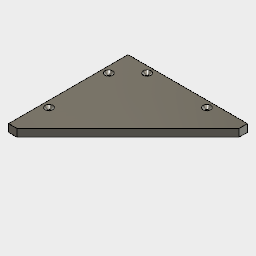
Full Assembly (Autodesk Fusion 360 archive; units mm, degrees)
design "Joining Plate (90 Degree)"
Autodesk Fusion 360 part; units mm, degrees
sketch "Sketch1" plane through (0, 0, 0) normal (0, 1, 0) x (1, 0, 0)
  line L0 (0, 0) -> (140, 0)
  line L1 (140, -10) -> (10, -140)
  line L2 (0, -140) -> (0, 0)
  line L3 (140, 0) -> (140, -10)
  line L4 (0, -140) -> (10, -140)
  circle A0 centre (30, -7.5) radius 1.5
  circle A1 centre (100, -7.5) radius 1.5
  circle A2 centre (7.5, -30) radius 1.5
  circle A3 centre (7.5, -100) radius 1.5
  dimension "d5" = 10
  dimension "d6" = 10
  dimension "d7" = 140
  dimension "d8" = 140
  dimension "d9" = 3
  dimension "d10" = 3
  dimension "d11" = 3
  dimension "d12" = 3
  dimension "d13" = 7.5
  dimension "d14" = 7.5
  dimension "d15" = 7.5
  dimension "d16" = 7.5
  dimension "d17" = 30
  dimension "d18" = 100
  dimension "d19" = 30
  dimension "d20" = 100
  measures "d5" distance of L0.end L1.start
  measures "d6" distance of L2.start L1.end
  measures "d7" distance of L0.start L2.start
  measures "d8" distance of L0.start L0.end
  measures "d9" diameter of A0
  measures "d10" diameter of A1
  measures "d11" diameter of A2
  measures "d12" diameter of A3
  measures "d13" distance of L0 A0.centre
  measures "d14" distance of L0 A1.centre
  measures "d15" distance of L2 A2.centre
  measures "d16" distance of L2 A3.centre
  measures "d17" distance of L0 A2.centre
  measures "d18" distance of L0 A3.centre
  measures "d19" distance of L2 A0.centre
  measures "d20" distance of L2 A1.centre
extrude "Extrude1" add sketch "Sketch1" along normal blind 9
chamfer "Chamfer1" distance 3 angle 45 4 edges at (28.6015, 9, 6.9576) (6.1015, 9, 29.4576) (98.6015, 9, 6.9576) (6.1015, 9, 99.4576)

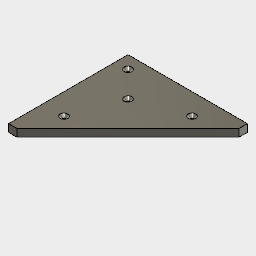
design "Joining Plate (180 Degree)"
Autodesk Fusion 360 part; units mm, degrees
sketch "Sketch1" plane through (0, 0, 0) normal (0, 1, 0) x (1, 0, 0)
  line L0 (0, 0) -> (140, 0)
  line L1 (140, -10) -> (10, -140)
  line L2 (0, -140) -> (0, 0)
  line L3 (140, 0) -> (140, -10)
  line L4 (0, -140) -> (10, -140)
  circle A0 centre (15, -15) radius 1.5
  circle A1 centre (100, -25) radius 1.5
  circle A2 centre (45, -45) radius 1.5
  circle A3 centre (25, -100) radius 1.5
  dimension "d5" = 10
  dimension "d6" = 10
  dimension "d7" = 140
  dimension "d8" = 140
  dimension "d9" = 3
  dimension "d10" = 3
  dimension "d11" = 3
  dimension "d12" = 3
  dimension "d26" = 45
  dimension "d27" = 45
  dimension "d28" = 15
  dimension "d29" = 15
  dimension "d30" = 25
  dimension "d31" = 25
  dimension "d32" = 100
  dimension "d33" = 100
  measures "d5" distance of L0.end L1.start
  measures "d6" distance of L2.start L1.end
  measures "d7" distance of L0.start L2.start
  measures "d8" distance of L0.start L0.end
  measures "d9" diameter of A0
  measures "d10" diameter of A1
  measures "d11" diameter of A2
  measures "d12" diameter of A3
  measures "d26" distance of L2 A2.centre
  measures "d27" distance of L0 A2.centre
  measures "d28" distance of L0 A0.centre
  measures "d29" distance of L2 A0.centre
  measures "d30" distance of L2 A3.centre
  measures "d31" distance of L0 A1.centre
  measures "d32" distance of L2 A1.centre
  measures "d33" distance of L0 A3.centre
extrude "Extrude1" add sketch "Sketch1" along normal blind 9
chamfer "Chamfer1" distance 3 angle 45 4 edges at (13.6015, 9, 14.4576) (43.6015, 9, 44.4576) (98.6015, 9, 24.4576) (23.6015, 9, 99.4576)

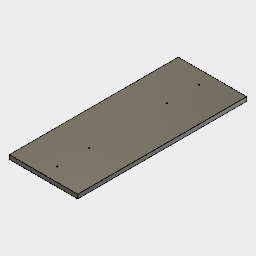
design "Gantry Foot Plate"
Autodesk Fusion 360 part; units mm, degrees
sketch "Sketch1" plane through (0, 0, 0) normal (0, 1, 0) x (1, 0, 0)
  line L0 (0, 0) -> (150, 0)
  line L1 (150, 0) -> (150, -370)
  line L2 (150, -370) -> (0, -370)
  line L3 (0, -370) -> (0, 0)
  line L4 (75, 0) -> (75, -370) construction
  circle A0 centre (75, -30) radius 1.5
  circle A1 centre (75, -100) radius 1.5
  circle A2 centre (75, -270) radius 1.5
  circle A3 centre (75, -340) radius 1.5
  dimension "d1" = 150
  dimension "d2" = 370
  dimension "d3" = 3
  dimension "d4" = 3
  dimension "d5" = 3
  dimension "d6" = 3
  dimension "d7" = 30
  dimension "d8" = 100
  dimension "d9" = 30
  dimension "d10" = 100
  measures "d1" distance of L0.start L0.end
  measures "d2" distance of L0.start L2.end
  measures "d3" diameter of A2
  measures "d4" diameter of A3
  measures "d5" diameter of A1
  measures "d6" diameter of A0
  measures "d7" distance of L0 A0.centre
  measures "d8" distance of L0 A1.centre
  measures "d9" distance of L2 A3.centre
  measures "d10" distance of L2 A2.centre
extrude "Extrude1" add sketch "Sketch1" along normal blind 9
chamfer "Chamfer1" distance 3 angle 45 4 edges at (73.6015, 0, 339.4576) (73.6015, 0, 269.4576) (73.6015, 0, 99.4576) (73.6015, 0, 29.4576)

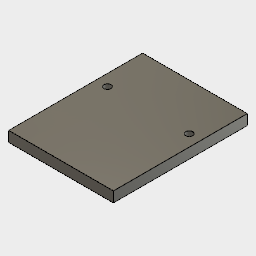
design "Gantry Mount Plate"
Autodesk Fusion 360 part; units mm, degrees
sketch "Sketch1" plane through (0, 0, 0) normal (0, 1, 0) x (1, 0, 0)
  line L0 (0, 0) -> (90, 0)
  line L1 (90, 0) -> (90, -115)
  line L2 (90, -115) -> (0, -115)
  line L3 (0, -115) -> (0, 0)
  dimension "d1" = 90
  dimension "d2" = 115
  measures "d1" distance of L0.start L0.end
  measures "d2" distance of L0.start L2.end
sketch "Sketch2" plane through (0, 0, 0) normal (0, 1, 0) x (1, 0, 0)
  circle A0 centre (10, -40) radius 3
  circle A1 centre (80, -40) radius 3
  line L0 (0, 0) -> (90, 0)
  line L1 (0, -115) -> (0, 0)
  line L2 (90, 0) -> (90, -115)
  dimension "d3" = 6
  dimension "d4" = 6
  dimension "d5" = 40
  dimension "d6" = 40
  dimension "d7" = 10
  dimension "d8" = 10
  measures "d3" diameter of A0
  measures "d4" diameter of A1
  measures "d5" distance of A0.centre L0
  measures "d6" distance of A1.centre L0
  measures "d7" distance of A0.centre L1
  measures "d8" distance of A1.centre L2
extrude "Extrude1" add sketch "Sketch1" along normal blind 9
extrude "Extrude2" cut sketch "Sketch2" along normal blind 9

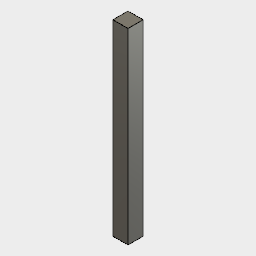
design "Gantry Base Beam"
Autodesk Fusion 360 part; units mm, degrees
sketch "Sketch1" plane through (0, 0, 0) normal (0, 1, 0) x (1, 0, 0)
  line L0 (0, 0) -> (30, 0)
  line L1 (30, 0) -> (30, -30)
  line L2 (30, -30) -> (0, -30)
  line L3 (0, -30) -> (0, 0)
  dimension "d1" = 30
  dimension "d2" = 30
  measures "d1" distance of L0.start L0.end
  measures "d2" distance of L0.start L2.end
extrude "Extrude1" add sketch "Sketch1" along normal blind 370

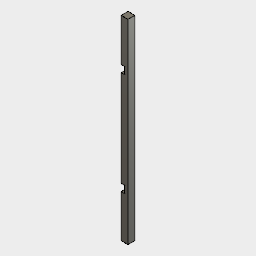
design "Frame Horizontal Beam"
Autodesk Fusion 360 part; units mm, degrees
sketch "Sketch1" plane through (0, 0, 0) normal (0, 1, 0) x (1, 0, 0)
  line L0 (0, 0) -> (30, 0)
  line L1 (30, 0) -> (30, -30)
  line L2 (30, -30) -> (0, -30)
  line L3 (0, -30) -> (0, 0)
  dimension "d1" = 30
  dimension "d2" = 30
  measures "d1" distance of L0.start L0.end
  measures "d2" distance of L0.start L2.end
extrude "Extrude1" add sketch "Sketch1" along normal blind 846
sketch "Sketch2" plane through (0, 0, 0) normal (-1, 0, 0) x (0, 0, 1)
  line L0 (0, 0) -> (30, 0)
  line L1 (30, 0) -> (30, 846)
  line L2 (30, 846) -> (0, 846)
  line L3 (0, 846) -> (0, 0)
  line L4 (0, 215) -> (30, 215)
  line L5 (30, 215) -> (30, 185)
  line L6 (30, 185) -> (0, 185)
  line L7 (0, 185) -> (0, 215)
  line L8 (0, 631) -> (30, 631)
  line L9 (30, 631) -> (30, 661)
  line L10 (30, 661) -> (0, 661)
  line L11 (0, 661) -> (0, 631)
  dimension "d5" = 30
  dimension "d6" = 30
  dimension "d7" = 185
  dimension "d8" = 185
  dimension "d9" = 380
  measures "d5" distance of L8.start L10.end
  measures "d6" distance of L4.end L5.end
  measures "d7" distance of L0 L6
  measures "d8" distance of L2 L10
extrude "Extrude2" cut sketch "Sketch2" against normal blind 15 contours L1 L3 L4 L5 L6 L7 | L1 L3 L8 L9 L10 L11

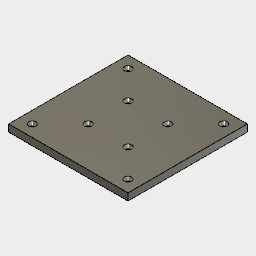
design "Joining Plate (360 Degrees)"
Autodesk Fusion 360 part; units mm, degrees
sketch "Sketch1" plane through (0, 0, 0) normal (0, 1, 0) x (1, 0, 0)
  line L0 (0, 0) -> (150, 0)
  line L1 (150, 0) -> (150, -150)
  line L2 (150, -150) -> (0, -150)
  line L3 (0, -150) -> (0, 0)
  circle A0 centre (15, -15) radius 1.5
  circle A1 centre (135, -15) radius 1.5
  circle A2 centre (135, -135) radius 1.5
  circle A3 centre (15, -135) radius 1.5
  circle A4 centre (50, -100) radius 1.5
  circle A5 centre (50, -50) radius 1.5
  circle A6 centre (100, -50) radius 1.5
  circle A7 centre (100, -100) radius 1.5
  dimension "d1" = 150
  dimension "d2" = 150
  dimension "d3" = 3
  dimension "d4" = 3
  dimension "d5" = 3
  dimension "d6" = 3
  dimension "d7" = 3
  dimension "d8" = 3
  dimension "d9" = 3
  dimension "d10" = 3
  dimension "d12" = 15
  dimension "d14" = 15
  dimension "d15" = 15
  dimension "d16" = 15
  dimension "d17" = 15
  dimension "d18" = 15
  dimension "d19" = 15
  dimension "d20" = 15
  dimension "d21" = 50
  dimension "d22" = 50
  dimension "d23" = 50
  dimension "d24" = 50
  dimension "d25" = 50
  dimension "d26" = 50
  dimension "d27" = 50
  dimension "d28" = 50
  measures "d1" distance of L0.start L0.end
  measures "d2" distance of L0.start L2.end
  measures "d3" diameter of A0
  measures "d4" diameter of A1
  measures "d5" diameter of A2
  measures "d6" diameter of A3
  measures "d7" diameter of A4
  measures "d8" diameter of A7
  measures "d9" diameter of A6
  measures "d10" diameter of A5
  measures "d12" distance of L3 A0.centre
  measures "d14" distance of L0 A0.centre
  measures "d15" distance of L1 A1.centre
  measures "d16" distance of L0 A1.centre
  measures "d17" distance of L1 A2.centre
  measures "d18" distance of L2 A2.centre
  measures "d19" distance of L3 A3.centre
  measures "d20" distance of L2 A3.centre
  measures "d21" distance of L3 A4.centre
  measures "d22" distance of L2 A4.centre
  measures "d23" distance of L2 A7.centre
  measures "d24" distance of L1 A7.centre
  measures "d25" distance of L0 A6.centre
  measures "d26" distance of L1 A6.centre
  measures "d27" distance of L3 A5.centre
  measures "d28" distance of L0 A5.centre
extrude "Extrude1" add sketch "Sketch1" along normal blind 9
chamfer "Chamfer1" distance 3 angle 45 8 edges at (13.6015, 9, 134.4576) (48.6015, 9, 99.4576) (98.6015, 9, 99.4576) (133.6015, 9, 134.4576) (133.6015, 9, 14.4576) (98.6015, 9, 49.4576) (48.6015, 9, 49.4576) (13.6015, 9, 14.4576)

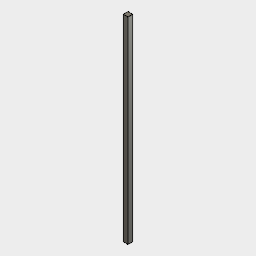
design "Gantry Top Beam"
Autodesk Fusion 360 part; units mm, degrees
sketch "Sketch1" plane through (0, 0, 0) normal (0, 1, 0) x (1, 0, 0)
  line L0 (0, 0) -> (30, 0)
  line L1 (30, 0) -> (30, -30)
  line L2 (30, -30) -> (0, -30)
  line L3 (0, -30) -> (0, 0)
  dimension "d1" = 30
  dimension "d2" = 30
  measures "d1" distance of L0.start L0.end
  measures "d2" distance of L0.start L2.end
extrude "Extrude1" add sketch "Sketch1" along normal blind 1224

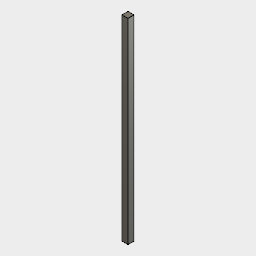
design "Gantry Side Beam"
Autodesk Fusion 360 part; units mm, degrees
sketch "Sketch1" plane through (0, 0, 0) normal (0, 1, 0) x (1, 0, 0)
  line L0 (0, 0) -> (30, 0)
  line L1 (30, 0) -> (30, -30)
  line L2 (30, -30) -> (0, -30)
  line L3 (0, -30) -> (0, 0)
  dimension "d1" = 30
  dimension "d2" = 30
  measures "d1" distance of L0.start L0.end
  measures "d2" distance of L0.start L2.end
extrude "Extrude1" add sketch "Sketch1" along normal blind 960

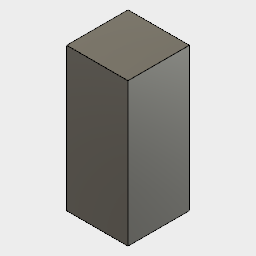
design "Gantry Mount Beam"
Autodesk Fusion 360 part; units mm, degrees
sketch "Sketch1" plane through (0, 0, 0) normal (0, 1, 0) x (1, 0, 0)
  line L0 (0, 0) -> (30, 0)
  line L1 (30, 0) -> (30, -30)
  line L2 (30, -30) -> (0, -30)
  line L3 (0, -30) -> (0, 0)
  dimension "d1" = 30
  dimension "d2" = 30
  measures "d1" distance of L0.start L0.end
  measures "d2" distance of L0.start L2.end
extrude "Extrude1" add sketch "Sketch1" along normal blind 70

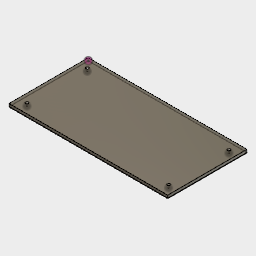
design "Projector Plate"
Autodesk Fusion 360 part; units mm, degrees
sketch "Sketch1" plane through (0, 0, 0) normal (0, 1, 0) x (1, 0, 0)
  line L0 (0, 0) -> (500, 0)
  line L1 (500, 0) -> (500, -250)
  line L2 (500, -250) -> (0, -250)
  line L3 (0, -250) -> (0, 0)
  circle A0 centre (27, -30) radius 1.5
  circle A1 centre (27, -220) radius 1.5
  circle A2 centre (473, -30) radius 1.5
  circle A3 centre (473, -220) radius 1.5
  dimension "d1" = 250
  dimension "d2" = 500
  dimension "d3" = 3
  dimension "d4" = 3
  dimension "d5" = 3
  dimension "d6" = 3
  dimension "d7" = 30
  dimension "d8" = 30
  dimension "d9" = 30
  dimension "d10" = 30
  dimension "d11" = 446
  dimension "d12" = 446
  dimension "d13" = 27
  dimension "d14" = 24
  dimension "d15" = 27
  measures "d1" distance of L0.end L1.end
  measures "d2" distance of L0.start L0.end
  measures "d3" diameter of A1
  measures "d4" diameter of A0
  measures "d5" diameter of A2
  measures "d6" diameter of A3
  measures "d7" distance of L0 A0.centre
  measures "d8" distance of L2 A1.centre
  measures "d9" distance of L2 A3.centre
  measures "d10" distance of L0 A2.centre
  measures "d11" distance of A0.centre A2.centre
  measures "d12" distance of A1.centre A3.centre
  measures "d13" distance of L3 A1.centre
  measures "d15" distance of L3 A0.centre
extrude "Extrude1" add sketch "Sketch1" along normal blind 9
chamfer "Chamfer1" distance 3 angle 45 4 edges at (25.6015, 9, 29.4576) (25.6015, 9, 219.4576) (471.6015, 9, 219.4576) (471.6015, 9, 29.4576)

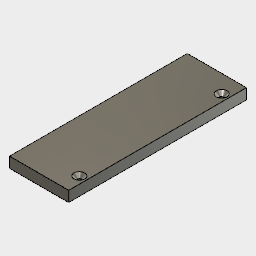
design "Driving Surface Support"
Autodesk Fusion 360 part; units mm, degrees
sketch "Sketch1" plane through (0, 0, 0) normal (0, 1, 0) x (1, 0, 0)
  line L0 (0, 0) -> (50, 0)
  line L1 (50, 0) -> (50, -150)
  line L2 (50, -150) -> (0, -150)
  line L3 (0, -150) -> (0, 0)
  circle A0 centre (44, -15) radius 1.5
  circle A1 centre (44, -135) radius 1.5
  dimension "d1" = 50
  dimension "d2" = 150
  dimension "d3" = 3
  dimension "d4" = 3
  dimension "d5" = 6
  dimension "d6" = 6
  dimension "d7" = 15
  dimension "d8" = 15
  measures "d1" distance of L0.start L0.end
  measures "d2" distance of L0.start L2.end
  measures "d3" diameter of A1
  measures "d4" diameter of A0
  measures "d5" distance of L1 A0.centre
  measures "d6" distance of L1 A1.centre
  measures "d7" distance of L2 A1.centre
  measures "d8" distance of L0 A0.centre
extrude "Extrude1" add sketch "Sketch1" along normal blind 9
chamfer "Chamfer1" distance 3 angle 45 2 edges at (42.6015, 9, 14.4576) (42.6015, 9, 134.4576)

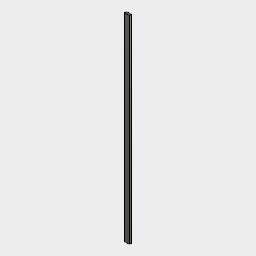
design "Edge Frame Horizontal"
Autodesk Fusion 360 part; units mm, degrees
sketch "Sketch1" plane through (0, 0, 0) normal (0, 1, 0) x (1, 0, 0)
  line L0 (0, 0) -> (30, 0)
  line L1 (30, 0) -> (30, -12)
  line L2 (30, -12) -> (0, -12)
  line L3 (0, -12) -> (0, 0)
  dimension "d1" = 30
  dimension "d2" = 12
  measures "d1" distance of L0.start L0.end
  measures "d2" distance of L0.end L1.end
extrude "Extrude1" add sketch "Sketch1" along normal blind 1200

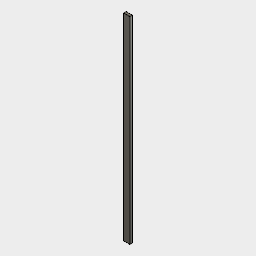
design "Edge Frame Vertical"
Autodesk Fusion 360 part; units mm, degrees
sketch "Sketch1" plane through (0, 0, 0) normal (0, 1, 0) x (1, 0, 0)
  line L0 (0, 0) -> (30, 0)
  line L1 (30, 0) -> (30, -12)
  line L2 (30, -12) -> (0, -12)
  line L3 (0, -12) -> (0, 0)
  dimension "d1" = 12
  dimension "d2" = 30
  measures "d1" distance of L0.end L1.end
  measures "d2" distance of L1.end L2.end
extrude "Extrude1" add sketch "Sketch1" along normal blind 924

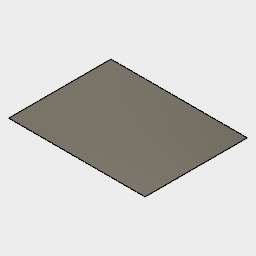
design "Driving Surface"
Autodesk Fusion 360 part; units mm, degrees
sketch "Sketch1" plane through (0, 0, 0) normal (0, 1, 0) x (1, 0, 0)
  line L0 (0, 0) -> (1200, 0)
  line L1 (1200, 0) -> (1200, -900)
  line L2 (1200, -900) -> (0, -900)
  line L3 (0, -900) -> (0, 0)
  dimension "d1" = 1200
  dimension "d2" = 900
  measures "d1" distance of L0.start L0.end
  measures "d2" distance of L0.start L2.end
extrude "Extrude1" add sketch "Sketch1" along normal blind 3

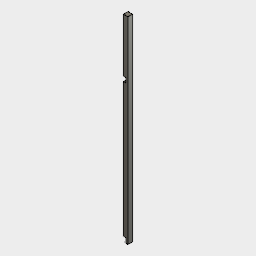
design "Frame Vertical Beam"
Autodesk Fusion 360 part; units mm, degrees
sketch "Sketch1" plane through (0, 0, 0) normal (0, 1, 0) x (1, 0, 0)
  line L0 (0, 0) -> (30, 0)
  line L1 (30, 0) -> (30, -30)
  line L2 (30, -30) -> (0, -30)
  line L3 (0, -30) -> (0, 0)
  dimension "d1" = 30
  dimension "d2" = 30
  measures "d1" distance of L0.start L0.end
  measures "d2" distance of L0.start L2.end
extrude "Extrude1" add sketch "Sketch1" along normal blind 1270
sketch "Sketch2" plane through (0, 0, 0) normal (-1, 0, 0) x (0, 0, 1)
  line L0 (0, 0) -> (30, 0)
  line L1 (30, 0) -> (30, 1270)
  line L2 (30, 1270) -> (0, 1270)
  line L3 (0, 1270) -> (0, 0)
  line L4 (0, 30) -> (30, 30)
  line L5 (30, 30) -> (30, 0)
  line L6 (30, 0) -> (0, 0)
  line L7 (0, 0) -> (0, 30)
  line L8 (0, 894) -> (30, 894)
  line L9 (30, 894) -> (30, 924)
  line L10 (30, 924) -> (0, 924)
  line L11 (0, 924) -> (0, 894)
  dimension "d5" = 30
  dimension "d6" = 30
  dimension "d12" = 924
  measures "d5" distance of L8.start L10.end
  measures "d6" distance of L4.end L0.end
  measures "d12" distance of L6 L10
extrude "Extrude2" cut sketch "Sketch2" against normal blind 15 contours L0 L1 L3 L4 L5 L6 L7 | L1 L3 L8 L9 L10 L11
